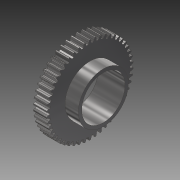
# Autodesk Inventor part: M-0.5 Zb-4mm M-0.7 Zb-5mm mN 21105000
Saved by Autodesk Inventor 2019.3 (Build 233278000, 278)
## iProperties
Created: 2018-08-17
Part Number: M-0.5 Zb-4mm M-0.7 Zb-5mm mN 21105000
Material: Stahl, Guss
Catalog Web Link: www.cadenas.de
Description: M-0.5 Zb-4mm M-0.7 Zb-5mm mN-Spur Gears, Steel, Module 0.5 and 0,7
Vendor: MAEDLER
Document SubType Name: Modeling
Designer: psadmin
Manufacturer: MAEDLER
Mass: 19 g
Surface Area: 18.1636 cm^2
Volume: 1.59221 cm^3
Density: 11.9331 g/cm^3
Appearance: Halbpoliert
Category: PARTsolutions
Company: MAEDLER
PSOL_IDENT_0: {$CADENAS_DATA\23d-libs\maedler\antriebselemente\stirnzahnraeder\stirnzahnraeder_stahl\modul_0.5_und
PSOL_IDENT_1: _0.7\m-0.5_zb-4mm_m-0.7_zb-5mm_mn.prj},237 {VTYP=3D},{NB=M-0.5 Zb-4mm M-0.7 Zb-5mm mN 21105000},{LIN
PSOL_IDENT_2: A=M-0.5 Zb-4mm M-0.7 Zb-5mm mN 21105000},{NN=M-0.5 Zb-4mm M-0.7 Zb-5mm mN},{DATE=27.10.2015 07:21:56
PSOL_IDENT_3: },{GEOMDATE=11.05.2009 09:51:00},{VERSION=},{LINEID=280},{WBVAR=},{WBNUMERIC=}  {NB=M-0.5 Zb-4mm M-0
PSOL_IDENT_4: .7 Zb-5mm mN 21105000},{LINA=M-0.5 Zb-4mm M-0.7 Zb-5mm mN 21105000},{KT=DUMMY},{ARTNR=21105000},{WST=
PSOL_IDENT_5: 11SMnPb30},{M=0.5},{Z=50},{PDF=PDF Katalogseite},{B1=4.0},{DA=26.00},{D=25.00},{NL=4},{ND=15},{B=5},
PSOL_IDENT_6: {MD=17.0},{GEW=19.000}
NN: M-0.5 Zb-4mm M-0.7 Zb-5mm mN
NT: Spur Gears, Steel, Module 0.5 and 0,7
NB: M-0.5 Zb-4mm M-0.7 Zb-5mm mN 21105000
NBSYN: M-0.5 Zb-4mm M-0.7 Zb-5mm mN $ARTNR.
LINA: M-0.5 Zb-4mm M-0.7 Zb-5mm mN 21105000
ARTNR: 21105000
WST: 11SMnPb30
M: 0.5
Z: 50
PDF: PDF Katalogseite
B1: 4
DA: 26
D: 25
NL: 4
ND: 15
B: 5
MD: 17
GEW: 19
SUPPLIER: MAEDLER
ARTICLENO: M-0.5 Zb-4mm M-0.7 Zb-5mm mN 21105000
BOMINFO: M-0.5 Zb-4mm M-0.7 Zb-5mm mN 21105000
CREATOR: CADENAS GmbH
Title: M-0.5 Zb-4mm M-0.7 Zb-5mm mN 21105000
Author: Cadenas PARTsolutions
Comments: Spur Gears, Steel, Module 0.5 and 0,7
Autodesk Inventor part; units mm, degrees
ref_plane "YZ Plane" through (0, 0, 0) normal (1, 0, 0) x (0, 1, 0)
ref_plane "XZ Plane" through (0, 0, 0) normal (0, 1, 0) x (-1, 0, 0)
ref_plane "XY Plane" through (0, 0, 0) normal (0, 0, 1) x (1, 0, 0)
sketch "Skizze_1" plane through (0, 0, 0) normal (1, 0, 0) x (0, 1, 0)
  arc A0 (0.1667, 12.9989) -> (-0.1667, 12.9989) centre (0, 0) ccw
  line L0 (-0.1667, 12.9989) -> (-0.3537, 12.495)
  line L1 (-0.3537, 12.495) -> (-0.5025, 11.9895)
  arc A1 (-0.5025, 11.9895) -> (-1.0041, 11.9579) centre (0, 0) ccw
  line L2 (-1.0041, 11.9579) -> (-1.2151, 12.4408)
  line L3 (-1.2151, 12.4408) -> (-1.4638, 12.9173)
  arc A2 (-1.4638, 12.9173) -> (-1.7946, 12.8755) centre (0, 0) ccw
  line L4 (-1.7946, 12.8755) -> (-1.917, 12.3521)
  line L5 (-1.917, 12.3521) -> (-2.0012, 11.832)
  arc A3 (-2.0012, 11.832) -> (-2.4949, 11.7378) centre (0, 0) ccw
  line L6 (-2.4949, 11.7378) -> (-2.7648, 12.1904)
  line L7 (-2.7648, 12.1904) -> (-3.0713, 12.632)
  arc A4 (-3.0713, 12.632) -> (-3.3941, 12.5491) centre (0, 0) ccw
  line L8 (-3.3941, 12.5491) -> (-3.45, 12.0145)
  line L9 (-3.45, 12.0145) -> (-3.4684, 11.4878)
  arc A5 (-3.4684, 11.4878) -> (-3.9464, 11.3325) centre (0, 0) ccw
  line L10 (-3.9464, 11.3325) -> (-4.2708, 11.7478)
  line L11 (-4.2708, 11.7478) -> (-4.6303, 12.1475)
  arc A6 (-4.6303, 12.1475) -> (-4.9402, 12.0247) centre (0, 0) ccw
  line L12 (-4.9402, 12.0247) -> (-4.9286, 11.4873)
  line L13 (-4.9286, 11.4873) -> (-4.8808, 10.9625)
  arc A7 (-4.8808, 10.9625) -> (-5.3356, 10.7485) centre (0, 0) ccw
  line L14 (-5.3356, 10.7485) -> (-5.7095, 11.1199)
  line L15 (-5.7095, 11.1199) -> (-6.1162, 11.4713)
  arc A8 (-6.1162, 11.4713) -> (-6.4083, 11.3108) centre (0, 0) ccw
  line L16 (-6.4083, 11.3108) -> (-6.3295, 10.779)
  line L17 (-6.3295, 10.779) -> (-6.2163, 10.2644)
  arc A9 (-6.2163, 10.2644) -> (-6.6407, 9.9951) centre (0, 0) ccw
  line L18 (-6.6407, 9.9951) -> (-7.0582, 10.3166)
  line L19 (-7.0582, 10.3166) -> (-7.5057, 10.6143)
  arc A10 (-7.5057, 10.6143) -> (-7.7754, 10.4184) centre (0, 0) ccw
  line L20 (-7.7754, 10.4184) -> (-7.6305, 9.9007)
  line L21 (-7.6305, 9.9007) -> (-7.4538, 9.4043)
  arc A11 (-7.4538, 9.4043) -> (-7.841, 9.0839) centre (0, 0) ccw
  line L22 (-7.841, 9.0839) -> (-8.2956, 9.3506)
  line L23 (-8.2956, 9.3506) -> (-8.7769, 9.5899)
  arc A12 (-8.7769, 9.5899) -> (-9.0199, 9.3617) centre (0, 0) ccw
  line L24 (-9.0199, 9.3617) -> (-8.8113, 8.8663)
  line L25 (-8.8113, 8.8663) -> (-8.5737, 8.396)
  arc A13 (-8.5737, 8.396) -> (-8.9177, 8.0296) centre (0, 0) ccw
  line L26 (-8.9177, 8.0296) -> (-9.4021, 8.2372)
  line L27 (-9.4021, 8.2372) -> (-9.9096, 8.4142)
  arc A14 (-9.9096, 8.4142) -> (-10.1221, 8.1574) centre (0, 0) ccw
  line L28 (-10.1221, 8.1574) -> (-9.853, 7.6921)
  line L29 (-9.853, 7.6921) -> (-9.5584, 7.2552)
  arc A15 (-9.5584, 7.2552) -> (-9.8538, 6.8486) centre (0, 0) ccw
  line L30 (-9.8538, 6.8486) -> (-10.3603, 6.9938)
  line L31 (-10.3603, 6.9938) -> (-10.8861, 7.1059)
  arc A16 (-10.8861, 7.1059) -> (-11.0647, 6.8245) centre (0, 0) ccw
  line L32 (-11.0647, 6.8245) -> (-10.7394, 6.3965)
  line L33 (-10.7394, 6.3965) -> (-10.3923, 6)
  arc A17 (-10.3923, 6) -> (-10.6344, 5.5596) centre (0, 0) ccw
  line L34 (-10.6344, 5.5596) -> (-11.1552, 5.6402)
  line L35 (-11.1552, 5.6402) -> (-11.6908, 5.6855)
  arc A18 (-11.6908, 5.6855) -> (-11.8327, 5.3839) centre (0, 0) ccw
  line L36 (-11.8327, 5.3839) -> (-11.4564, 5)
  line L37 (-11.4564, 5) -> (-11.0624, 4.6502)
  arc A19 (-11.0624, 4.6502) -> (-11.2474, 4.1829) centre (0, 0) ccw
  line L38 (-11.2474, 4.1829) -> (-11.7741, 4.1976)
  line L39 (-11.7741, 4.1976) -> (-12.3112, 4.1754)
  arc A20 (-12.3112, 4.1754) -> (-12.4142, 3.8584) centre (0, 0) ccw
  line L40 (-12.4142, 3.8584) -> (-11.9928, 3.5248)
  line L41 (-11.9928, 3.5248) -> (-11.558, 3.227)
  arc A21 (-11.558, 3.227) -> (-11.6829, 2.7402) centre (0, 0) ccw
  line L42 (-11.6829, 2.7402) -> (-12.2074, 2.6888)
  line L43 (-12.2074, 2.6888) -> (-12.7375, 2.5995)
  arc A22 (-12.7375, 2.5995) -> (-12.7999, 2.272) centre (0, 0) ccw
  line L44 (-12.7999, 2.272) -> (-12.34, 1.9939)
  line L45 (-12.34, 1.9939) -> (-11.8713, 1.753)
  arc A23 (-11.8713, 1.753) -> (-11.9343, 1.2543) centre (0, 0) ccw
  line L46 (-11.9343, 1.2543) -> (-12.4481, 1.1376)
  line L47 (-12.4481, 1.1376) -> (-12.9628, 0.9825)
  arc A24 (-12.9628, 0.9825) -> (-12.9837, 0.6499) centre (0, 0) ccw
  line L48 (-12.9837, 0.6499) -> (-12.4925, 0.4315)
  line L49 (-12.4925, 0.4315) -> (-11.9974, 0.2513)
  arc A25 (-11.9974, 0.2513) -> (-11.9974, -0.2513) centre (0, 0) ccw
  line L50 (-11.9974, -0.2513) -> (-12.4925, -0.4315)
  line L51 (-12.4925, -0.4315) -> (-12.9837, -0.6499)
  arc A26 (-12.9837, -0.6499) -> (-12.9628, -0.9825) centre (0, 0) ccw
  line L52 (-12.9628, -0.9825) -> (-12.4481, -1.1376)
  line L53 (-12.4481, -1.1376) -> (-11.9343, -1.2543)
  arc A27 (-11.9343, -1.2543) -> (-11.8713, -1.753) centre (0, 0) ccw
  line L54 (-11.8713, -1.753) -> (-12.34, -1.9939)
  line L55 (-12.34, -1.9939) -> (-12.7999, -2.272)
  arc A28 (-12.7999, -2.272) -> (-12.7375, -2.5995) centre (0, 0) ccw
  line L56 (-12.7375, -2.5995) -> (-12.2074, -2.6888)
  line L57 (-12.2074, -2.6888) -> (-11.6829, -2.7402)
  arc A29 (-11.6829, -2.7402) -> (-11.558, -3.227) centre (0, 0) ccw
  line L58 (-11.558, -3.227) -> (-11.9928, -3.5248)
  line L59 (-11.9928, -3.5248) -> (-12.4142, -3.8584)
  arc A30 (-12.4142, -3.8584) -> (-12.3112, -4.1754) centre (0, 0) ccw
  line L60 (-12.3112, -4.1754) -> (-11.7741, -4.1976)
  line L61 (-11.7741, -4.1976) -> (-11.2474, -4.1829)
  arc A31 (-11.2474, -4.1829) -> (-11.0624, -4.6502) centre (0, 0) ccw
  line L62 (-11.0624, -4.6502) -> (-11.4564, -5)
  line L63 (-11.4564, -5) -> (-11.8327, -5.3839)
  arc A32 (-11.8327, -5.3839) -> (-11.6908, -5.6855) centre (0, 0) ccw
  line L64 (-11.6908, -5.6855) -> (-11.1552, -5.6402)
  line L65 (-11.1552, -5.6402) -> (-10.6344, -5.5596)
  arc A33 (-10.6344, -5.5596) -> (-10.3923, -6) centre (0, 0) ccw
  line L66 (-10.3923, -6) -> (-10.7394, -6.3965)
  line L67 (-10.7394, -6.3965) -> (-11.0647, -6.8245)
  arc A34 (-11.0647, -6.8245) -> (-10.8861, -7.1059) centre (0, 0) ccw
  line L68 (-10.8861, -7.1059) -> (-10.3603, -6.9938)
  line L69 (-10.3603, -6.9938) -> (-9.8538, -6.8486)
  arc A35 (-9.8538, -6.8486) -> (-9.5584, -7.2552) centre (0, 0) ccw
  line L70 (-9.5584, -7.2552) -> (-9.853, -7.6921)
  line L71 (-9.853, -7.6921) -> (-10.1221, -8.1574)
  arc A36 (-10.1221, -8.1574) -> (-9.9096, -8.4142) centre (0, 0) ccw
  line L72 (-9.9096, -8.4142) -> (-9.4021, -8.2372)
  line L73 (-9.4021, -8.2372) -> (-8.9177, -8.0296)
  arc A37 (-8.9177, -8.0296) -> (-8.5737, -8.396) centre (0, 0) ccw
  line L74 (-8.5737, -8.396) -> (-8.8113, -8.8663)
  line L75 (-8.8113, -8.8663) -> (-9.0199, -9.3617)
  arc A38 (-9.0199, -9.3617) -> (-8.7769, -9.5899) centre (0, 0) ccw
  line L76 (-8.7769, -9.5899) -> (-8.2956, -9.3506)
  line L77 (-8.2956, -9.3506) -> (-7.841, -9.0839)
  arc A39 (-7.841, -9.0839) -> (-7.4538, -9.4043) centre (0, 0) ccw
  line L78 (-7.4538, -9.4043) -> (-7.6305, -9.9007)
  line L79 (-7.6305, -9.9007) -> (-7.7754, -10.4184)
  arc A40 (-7.7754, -10.4184) -> (-7.5057, -10.6143) centre (0, 0) ccw
  line L80 (-7.5057, -10.6143) -> (-7.0582, -10.3166)
  line L81 (-7.0582, -10.3166) -> (-6.6407, -9.9951)
  arc A41 (-6.6407, -9.9951) -> (-6.2163, -10.2644) centre (0, 0) ccw
  line L82 (-6.2163, -10.2644) -> (-6.3295, -10.779)
  line L83 (-6.3295, -10.779) -> (-6.4083, -11.3108)
  arc A42 (-6.4083, -11.3108) -> (-6.1162, -11.4713) centre (0, 0) ccw
  line L84 (-6.1162, -11.4713) -> (-5.7095, -11.1199)
  line L85 (-5.7095, -11.1199) -> (-5.3356, -10.7485)
  arc A43 (-5.3356, -10.7485) -> (-4.8808, -10.9625) centre (0, 0) ccw
  line L86 (-4.8808, -10.9625) -> (-4.9286, -11.4873)
  line L87 (-4.9286, -11.4873) -> (-4.9402, -12.0247)
  arc A44 (-4.9402, -12.0247) -> (-4.6303, -12.1475) centre (0, 0) ccw
  line L88 (-4.6303, -12.1475) -> (-4.2708, -11.7478)
  line L89 (-4.2708, -11.7478) -> (-3.9464, -11.3325)
  arc A45 (-3.9464, -11.3325) -> (-3.4684, -11.4878) centre (0, 0) ccw
  line L90 (-3.4684, -11.4878) -> (-3.45, -12.0145)
  line L91 (-3.45, -12.0145) -> (-3.3941, -12.5491)
  arc A46 (-3.3941, -12.5491) -> (-3.0713, -12.632) centre (0, 0) ccw
  line L92 (-3.0713, -12.632) -> (-2.7648, -12.1904)
  line L93 (-2.7648, -12.1904) -> (-2.4949, -11.7378)
  arc A47 (-2.4949, -11.7378) -> (-2.0012, -11.832) centre (0, 0) ccw
  line L94 (-2.0012, -11.832) -> (-1.917, -12.3521)
  line L95 (-1.917, -12.3521) -> (-1.7946, -12.8755)
  arc A48 (-1.7946, -12.8755) -> (-1.4638, -12.9173) centre (0, 0) ccw
  line L96 (-1.4638, -12.9173) -> (-1.2151, -12.4408)
  line L97 (-1.2151, -12.4408) -> (-1.0041, -11.9579)
  arc A49 (-1.0041, -11.9579) -> (-0.5025, -11.9895) centre (0, 0) ccw
  line L98 (-0.5025, -11.9895) -> (-0.3537, -12.495)
  line L99 (-0.3537, -12.495) -> (-0.1667, -12.9989)
  arc A50 (-0.1667, -12.9989) -> (0.1667, -12.9989) centre (0, 0) ccw
  line L100 (0.1667, -12.9989) -> (0.3537, -12.495)
  line L101 (0.3537, -12.495) -> (0.5025, -11.9895)
  arc A51 (0.5025, -11.9895) -> (1.0041, -11.9579) centre (0, 0) ccw
  line L102 (1.0041, -11.9579) -> (1.2151, -12.4408)
  line L103 (1.2151, -12.4408) -> (1.4638, -12.9173)
  arc A52 (1.4638, -12.9173) -> (1.7946, -12.8755) centre (0, 0) ccw
  line L104 (1.7946, -12.8755) -> (1.917, -12.3521)
  line L105 (1.917, -12.3521) -> (2.0012, -11.832)
  arc A53 (2.0012, -11.832) -> (2.4949, -11.7378) centre (0, 0) ccw
  line L106 (2.4949, -11.7378) -> (2.7648, -12.1904)
  line L107 (2.7648, -12.1904) -> (3.0713, -12.632)
  arc A54 (3.0713, -12.632) -> (3.3941, -12.5491) centre (0, 0) ccw
  line L108 (3.3941, -12.5491) -> (3.45, -12.0145)
  line L109 (3.45, -12.0145) -> (3.4684, -11.4878)
  arc A55 (3.4684, -11.4878) -> (3.9464, -11.3325) centre (0, 0) ccw
  line L110 (3.9464, -11.3325) -> (4.2708, -11.7478)
  line L111 (4.2708, -11.7478) -> (4.6303, -12.1475)
  arc A56 (4.6303, -12.1475) -> (4.9402, -12.0247) centre (0, 0) ccw
  line L112 (4.9402, -12.0247) -> (4.9286, -11.4873)
  line L113 (4.9286, -11.4873) -> (4.8808, -10.9625)
  arc A57 (4.8808, -10.9625) -> (5.3356, -10.7485) centre (0, 0) ccw
  line L114 (5.3356, -10.7485) -> (5.7095, -11.1199)
  line L115 (5.7095, -11.1199) -> (6.1162, -11.4713)
  arc A58 (6.1162, -11.4713) -> (6.4083, -11.3108) centre (0, 0) ccw
  line L116 (6.4083, -11.3108) -> (6.3295, -10.779)
  line L117 (6.3295, -10.779) -> (6.2163, -10.2644)
  arc A59 (6.2163, -10.2644) -> (6.6407, -9.9951) centre (0, 0) ccw
  line L118 (6.6407, -9.9951) -> (7.0582, -10.3166)
  line L119 (7.0582, -10.3166) -> (7.5057, -10.6143)
  arc A60 (7.5057, -10.6143) -> (7.7754, -10.4184) centre (0, 0) ccw
  line L120 (7.7754, -10.4184) -> (7.6305, -9.9007)
  line L121 (7.6305, -9.9007) -> (7.4538, -9.4043)
  arc A61 (7.4538, -9.4043) -> (7.841, -9.0839) centre (0, 0) ccw
  line L122 (7.841, -9.0839) -> (8.2956, -9.3506)
  line L123 (8.2956, -9.3506) -> (8.7769, -9.5899)
  arc A62 (8.7769, -9.5899) -> (9.0199, -9.3617) centre (0, 0) ccw
  line L124 (9.0199, -9.3617) -> (8.8113, -8.8663)
  line L125 (8.8113, -8.8663) -> (8.5737, -8.396)
  arc A63 (8.5737, -8.396) -> (8.9177, -8.0296) centre (0, 0) ccw
  line L126 (8.9177, -8.0296) -> (9.4021, -8.2372)
  line L127 (9.4021, -8.2372) -> (9.9096, -8.4142)
  arc A64 (9.9096, -8.4142) -> (10.1221, -8.1574) centre (0, 0) ccw
  line L128 (10.1221, -8.1574) -> (9.853, -7.6921)
  line L129 (9.853, -7.6921) -> (9.5584, -7.2552)
  arc A65 (9.5584, -7.2552) -> (9.8538, -6.8486) centre (0, 0) ccw
  line L130 (9.8538, -6.8486) -> (10.3603, -6.9938)
  line L131 (10.3603, -6.9938) -> (10.8861, -7.1059)
  arc A66 (10.8861, -7.1059) -> (11.0647, -6.8245) centre (0, 0) ccw
  line L132 (11.0647, -6.8245) -> (10.7394, -6.3965)
  line L133 (10.7394, -6.3965) -> (10.3923, -6)
  arc A67 (10.3923, -6) -> (10.6344, -5.5596) centre (0, 0) ccw
  line L134 (10.6344, -5.5596) -> (11.1552, -5.6402)
  line L135 (11.1552, -5.6402) -> (11.6908, -5.6855)
  arc A68 (11.6908, -5.6855) -> (11.8327, -5.3839) centre (0, 0) ccw
  line L136 (11.8327, -5.3839) -> (11.4564, -5)
  line L137 (11.4564, -5) -> (11.0624, -4.6502)
  arc A69 (11.0624, -4.6502) -> (11.2474, -4.1829) centre (0, 0) ccw
  line L138 (11.2474, -4.1829) -> (11.7741, -4.1976)
  line L139 (11.7741, -4.1976) -> (12.3112, -4.1754)
  arc A70 (12.3112, -4.1754) -> (12.4142, -3.8584) centre (0, 0) ccw
  line L140 (12.4142, -3.8584) -> (11.9928, -3.5248)
  line L141 (11.9928, -3.5248) -> (11.558, -3.227)
  arc A71 (11.558, -3.227) -> (11.6829, -2.7402) centre (0, 0) ccw
  line L142 (11.6829, -2.7402) -> (12.2074, -2.6888)
  line L143 (12.2074, -2.6888) -> (12.7375, -2.5995)
  arc A72 (12.7375, -2.5995) -> (12.7999, -2.272) centre (0, 0) ccw
  line L144 (12.7999, -2.272) -> (12.34, -1.9939)
  line L145 (12.34, -1.9939) -> (11.8713, -1.753)
  arc A73 (11.8713, -1.753) -> (11.9343, -1.2543) centre (0, 0) ccw
  line L146 (11.9343, -1.2543) -> (12.4481, -1.1376)
  line L147 (12.4481, -1.1376) -> (12.9628, -0.9825)
  arc A74 (12.9628, -0.9825) -> (12.9837, -0.6499) centre (0, 0) ccw
  line L148 (12.9837, -0.6499) -> (12.4925, -0.4315)
  line L149 (12.4925, -0.4315) -> (11.9974, -0.2513)
  arc A75 (11.9974, -0.2513) -> (11.9974, 0.2513) centre (0, 0) ccw
  line L150 (11.9974, 0.2513) -> (12.4925, 0.4315)
  line L151 (12.4925, 0.4315) -> (12.9837, 0.6499)
  arc A76 (12.9837, 0.6499) -> (12.9628, 0.9825) centre (0, 0) ccw
  line L152 (12.9628, 0.9825) -> (12.4481, 1.1376)
  line L153 (12.4481, 1.1376) -> (11.9343, 1.2543)
  arc A77 (11.9343, 1.2543) -> (11.8713, 1.753) centre (0, 0) ccw
  line L154 (11.8713, 1.753) -> (12.34, 1.9939)
  line L155 (12.34, 1.9939) -> (12.7999, 2.272)
  arc A78 (12.7999, 2.272) -> (12.7375, 2.5995) centre (0, 0) ccw
  line L156 (12.7375, 2.5995) -> (12.2074, 2.6888)
  line L157 (12.2074, 2.6888) -> (11.6829, 2.7402)
  arc A79 (11.6829, 2.7402) -> (11.558, 3.227) centre (0, 0) ccw
  line L158 (11.558, 3.227) -> (11.9928, 3.5248)
  line L159 (11.9928, 3.5248) -> (12.4142, 3.8584)
  arc A80 (12.4142, 3.8584) -> (12.3112, 4.1754) centre (0, 0) ccw
  line L160 (12.3112, 4.1754) -> (11.7741, 4.1976)
  line L161 (11.7741, 4.1976) -> (11.2474, 4.1829)
  arc A81 (11.2474, 4.1829) -> (11.0624, 4.6502) centre (0, 0) ccw
  line L162 (11.0624, 4.6502) -> (11.4564, 5)
  line L163 (11.4564, 5) -> (11.8327, 5.3839)
  arc A82 (11.8327, 5.3839) -> (11.6908, 5.6855) centre (0, 0) ccw
  line L164 (11.6908, 5.6855) -> (11.1552, 5.6402)
  line L165 (11.1552, 5.6402) -> (10.6344, 5.5596)
  arc A83 (10.6344, 5.5596) -> (10.3923, 6) centre (0, 0) ccw
  line L166 (10.3923, 6) -> (10.7394, 6.3965)
  line L167 (10.7394, 6.3965) -> (11.0647, 6.8245)
  arc A84 (11.0647, 6.8245) -> (10.8861, 7.1059) centre (0, 0) ccw
  line L168 (10.8861, 7.1059) -> (10.3603, 6.9938)
  line L169 (10.3603, 6.9938) -> (9.8538, 6.8486)
  arc A85 (9.8538, 6.8486) -> (9.5584, 7.2552) centre (0, 0) ccw
  line L170 (9.5584, 7.2552) -> (9.853, 7.6921)
  line L171 (9.853, 7.6921) -> (10.1221, 8.1574)
  arc A86 (10.1221, 8.1574) -> (9.9096, 8.4142) centre (0, 0) ccw
  line L172 (9.9096, 8.4142) -> (9.4021, 8.2372)
  line L173 (9.4021, 8.2372) -> (8.9177, 8.0296)
  arc A87 (8.9177, 8.0296) -> (8.5737, 8.396) centre (0, 0) ccw
  line L174 (8.5737, 8.396) -> (8.8113, 8.8663)
  line L175 (8.8113, 8.8663) -> (9.0199, 9.3617)
  arc A88 (9.0199, 9.3617) -> (8.7769, 9.5899) centre (0, 0) ccw
  line L176 (8.7769, 9.5899) -> (8.2956, 9.3506)
  line L177 (8.2956, 9.3506) -> (7.841, 9.0839)
  arc A89 (7.841, 9.0839) -> (7.4538, 9.4043) centre (0, 0) ccw
  line L178 (7.4538, 9.4043) -> (7.6305, 9.9007)
  line L179 (7.6305, 9.9007) -> (7.7754, 10.4184)
  arc A90 (7.7754, 10.4184) -> (7.5057, 10.6143) centre (0, 0) ccw
  line L180 (7.5057, 10.6143) -> (7.0582, 10.3166)
  line L181 (7.0582, 10.3166) -> (6.6407, 9.9951)
  arc A91 (6.6407, 9.9951) -> (6.2163, 10.2644) centre (0, 0) ccw
  line L182 (6.2163, 10.2644) -> (6.3295, 10.779)
  line L183 (6.3295, 10.779) -> (6.4083, 11.3108)
  arc A92 (6.4083, 11.3108) -> (6.1162, 11.4713) centre (0, 0) ccw
  line L184 (6.1162, 11.4713) -> (5.7095, 11.1199)
  line L185 (5.7095, 11.1199) -> (5.3356, 10.7485)
  arc A93 (5.3356, 10.7485) -> (4.8808, 10.9625) centre (0, 0) ccw
  line L186 (4.8808, 10.9625) -> (4.9286, 11.4873)
  line L187 (4.9286, 11.4873) -> (4.9402, 12.0247)
  arc A94 (4.9402, 12.0247) -> (4.6303, 12.1475) centre (0, 0) ccw
  line L188 (4.6303, 12.1475) -> (4.2708, 11.7478)
  line L189 (4.2708, 11.7478) -> (3.9464, 11.3325)
  arc A95 (3.9464, 11.3325) -> (3.4684, 11.4878) centre (0, 0) ccw
  line L190 (3.4684, 11.4878) -> (3.45, 12.0145)
  line L191 (3.45, 12.0145) -> (3.3941, 12.5491)
  arc A96 (3.3941, 12.5491) -> (3.0713, 12.632) centre (0, 0) ccw
  line L192 (3.0713, 12.632) -> (2.7648, 12.1904)
  line L193 (2.7648, 12.1904) -> (2.4949, 11.7378)
  arc A97 (2.4949, 11.7378) -> (2.0012, 11.832) centre (0, 0) ccw
  line L194 (2.0012, 11.832) -> (1.917, 12.3521)
  line L195 (1.917, 12.3521) -> (1.7946, 12.8755)
  arc A98 (1.7946, 12.8755) -> (1.4638, 12.9173) centre (0, 0) ccw
  line L196 (1.4638, 12.9173) -> (1.2151, 12.4408)
  line L197 (1.2151, 12.4408) -> (1.0041, 11.9579)
  arc A99 (1.0041, 11.9579) -> (0.5025, 11.9895) centre (0, 0) ccw
  line L198 (0.5025, 11.9895) -> (0.3537, 12.495)
  line L199 (0.3537, 12.495) -> (0.1667, 12.9989)
  constraints: 400 end point, 200 point on circle, 100 centre point
extrude "Extrusion1" add sketch "Skizze_1" along normal mid plane 4
sketch "Skizze_2" plane through (0, 0, 0) normal (0, 0, 1) x (1, 0, 0)
  line L0 (6, 0) -> (2, 0)
  line L1 (2, 0) -> (2, 7.5)
  line L2 (2, 7.5) -> (6, 7.5)
  line L3 (6, 7.5) -> (6, 0)
  line L4 (6, 0) -> (2, 0)
  constraints: 10 end point
revolve "Revolution1" add sketch "Skizze_2" angle 360 about axis through (6, 0, 0) along (1, 0, 0)
sketch "Skizze_3" plane through (6, 0, 0) normal (1, 0, 0) x (0, 1, 0)
  circle A0 centre (0, 0) radius 2.5
  constraints: 1 centre point
extrude "Extrusion2" cut sketch "Skizze_3" along normal mid plane 16
sketch "Skizze4" plane through (-2, 0, 0) normal (-1, 0, 0) x (0, 0, 1)
  circle A0 centre (0, 0) radius 6.5
  dimension "d5" = 13
  constraints: 1 centre point, 1 coincident
  measures "d5" diameter of A0
extrude "Extrusion3" cut sketch "Skizze4" against normal through all
body "Solid1"
